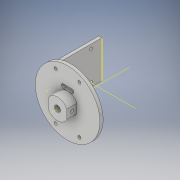
# Autodesk Inventor part: LidarLiteV3Mount
Saved by Autodesk Inventor 2019 (Build 230136000, 136)
## iProperties
Created: 2018-05-20
Part Number: LidarLiteV3Mount
Material: Generic
Document SubType Name: Modeling
Designer: samps
Density: 1 g/cm^3
Appearance: Default
Author: samps
Autodesk Inventor part; units mm, degrees
ref_plane "YZ Plane" through (0, 0, 0) normal (1, 0, 0) x (0, 1, 0)
ref_plane "XZ Plane" through (0, 0, 0) normal (0, 1, 0) x (-1, 0, 0)
ref_plane "XY Plane" through (0, 0, 0) normal (0, 0, 1) x (1, 0, 0)
sketch "Sketch1" plane through (0, 0, 0) normal (0, 0, 1) x (1, 0, 0)
  circle A0 centre (0, 0) radius 10
  dimension "d0" = 20
  constraints: 1 centre point, 1 coincident
  measures "d0" diameter of A0
extrude "Extrusion1" add sketch "Sketch1" along normal blind 10
sketch "Sketch2" plane through (0, 0, 10) normal (0, 0, 1) x (1, 0, 0)
  point P0 (0, 0)
  point P1 (0, 0)
  constraints: 1 coincident
hole "Hole1" at (0, 0, 10) direction (0, 0, -1) diameter 5 end through all
chamfer "Chamfer1" distance 0.5 angle 45 1 edges at (0, 2.5, 10)
sketch "Sketch3" plane through (0, 0, 10) normal (0, 0, 1) x (1, 0, 0)
  circle A0 centre (0, 0) radius 10 projected
  line L0 (-10, 0) -> (-9, 0)
  line L1 (-9, 0) -> (-9, 4.3589)
  line L2 (-9, 4.3589) -> (-10, 4.3589)
  line L3 (-10, 4.3589) -> (-10, 0)
  line L4 (-10, 0) -> (-9, 0)
  line L5 (-9, 0) -> (-9, -4.4002)
  line L6 (-9, -4.4002) -> (-10, -4.4002)
  line L7 (-10, -4.4002) -> (-10, 0)
  line L8 (10.026, 0) -> (9.026, 0)
  line L9 (9.026, 0) -> (9.026, 4.3589)
  line L10 (9.026, 4.3589) -> (10.026, 4.3589)
  line L11 (10.026, 4.3589) -> (10.026, 0)
  line L12 (10.026, 0) -> (9.026, 0)
  line L13 (9.026, 0) -> (9.026, -4.4002)
  line L14 (9.026, -4.4002) -> (10.026, -4.4002)
  line L15 (10.026, -4.4002) -> (10.026, 0)
  dimension "d13" = 1
  dimension "d14" = 1
  dimension "d15" = 1
  constraints: 32 end point, 8 parallel, 4 horizontal, 4 perpendicular, 4 point on line, 2 point on circle
  measures "d13" distance of L2.end L1.end
  measures "d14" distance of L5.end L6.end
  measures "d15" distance of L9.end L10.end
extrude "Extrusion2" cut sketch "Sketch3" against normal blind 10 contours L1 L0 A0 | L0 L5 A0 | A0 L5 L6 L7 | L9 L10 L11 L8 A0 | A0 L8 L9 | L8 L15 L14 L13 A0 | A0 L13 L8
sketch "Sketch4" plane through (9.026, -4.3048, 10) normal (1, 0, 0) x (0, 0, -1)
  line L0 (10, 4.3048) -> (5, 4.3048)
  line L1 (0.5, 1.8048) -> (0.5, 6.8048) projected
  dimension "d18" = 5
  constraints: 2 end point, 1 perpendicular
  measures "d18" distance of L0.start L0.end
hole "Hole2" at (9.026, 0, 5) direction (-1, 0, 0) diameter 3 end through all
sketch "Sketch5" plane through (9.026, -4.3048, 10) normal (1, 0, 0) x (0, 0, -1)
  circle A0 centre (5, 4.3048) radius 1.5 projected
  point P0 (10, 4.3048)
  constraints: 1 coincident
hole "Hole3" at (9.026, 0, 5) direction (-1, 0, 0) diameter 3.5 depth 3.5
sketch "Sketch6" plane through (-9, -4.3589, 10) normal (-1, 0, 0) x (0, 0, 1)
  circle A0 centre (-5, 4.3589) radius 1.5 projected
  point P0 (-10, 4.3589)
  constraints: 1 coincident
hole "Hole4" at (-9, 0, 5) direction (1, 0, 0) diameter 3.5 depth 3.5
sketch "Sketch7" plane through (0, 0, 0) normal (0, 0, -1) x (-1, 0, 0)
  line L0 (0, 0) -> (-9.026, 0)
  line L1 (-9.026, 0) -> (-9.026, 18)
  line L2 (-9.026, 18) -> (0, 18)
  line L3 (0, 18) -> (0, 0)
  line L4 (0, 0) -> (-9.026, 0)
  line L5 (-9.026, 0) -> (-9.026, -18)
  line L6 (-9.026, -18) -> (0, -18)
  line L7 (0, -18) -> (0, 0)
  line L8 (0, 18) -> (23, 18)
  line L9 (23, 18) -> (23, -18)
  line L10 (23, -18) -> (0, -18)
  line L11 (0, -18) -> (0, 18)
  dimension "d40" = 9.026
  dimension "d41" = 18
  dimension "d42" = 18
  dimension "d43" = 23
  constraints: 24 end point, 6 parallel, 3 horizontal, 3 perpendicular, 2 point on line
  measures "d40" distance of L1.end L2.end
  measures "d41" distance of L0.end L1.end
  measures "d42" distance of L5.end L4.end
  measures "d43" distance of L9.end L10.end
extrude "Extrusion3" add sketch "Sketch7" along normal blind 3
sketch "Sketch8" plane through (0, 0, -3) normal (0, 0, -1) x (-1, 0, 0)
  line L0 (23, 18) -> (-9.026, 18) projected
  line L1 (-9.026, -18) -> (23, -18) projected
  line L2 (23, 18) -> (20, 18)
  line L3 (20, 18) -> (20, -18)
  line L4 (20, -18) -> (23, -18)
  line L5 (23, -18) -> (23, 18)
  point P0 (0, 0)
  dimension "d46" = 3
  constraints: 8 end point, 2 parallel, 1 horizontal, 1 perpendicular, 1 point on line
  measures "d46" distance of L4.end L3.end
extrude "Extrusion4" add sketch "Sketch8" along normal blind 50
sketch "Sketch9" plane through (-20, -18, -3) normal (1, 0, 0) x (0, 0, -1)
  line L0 (0, 0) -> (0, 36) projected
  line L1 (0, 36) -> (25, 36)
  line L2 (-3, 36) -> (50, 36) projected
  line L3 (25, 36) -> (25, 18)
  line L4 (-3, 0) -> (50, 0) projected
  line L5 (25, 18) -> (39.5, 18)
  line L6 (39.5, 18) -> (39.5, 31.9)
  line L7 (39.5, 31.9) -> (25, 31.9)
  line L8 (25, 31.9) -> (25, 18)
  line L9 (25, 18) -> (39.5, 18)
  line L10 (39.5, 18) -> (39.5, 4.1)
  line L11 (39.5, 4.1) -> (25, 4.1)
  line L12 (25, 4.1) -> (25, 18)
  line L13 (25, 18) -> (10.5, 18)
  line L14 (10.5, 18) -> (10.5, 31.9)
  line L15 (10.5, 31.9) -> (25, 31.9)
  line L16 (25, 31.9) -> (25, 18)
  line L17 (25, 18) -> (10.5, 18)
  line L18 (10.5, 18) -> (10.5, 4.1)
  line L19 (10.5, 4.1) -> (25, 4.1)
  line L20 (25, 4.1) -> (25, 18)
  point P0 (-3, 18)
  dimension "d49" = 25
  dimension "d50" = 18
  dimension "d51" = 14.5
  dimension "d52" = 13.9
  dimension "d53" = 13.9
  dimension "d54" = 14.5
  constraints: 36 end point, 8 parallel, 5 perpendicular, 5 point on line, 4 horizontal
  measures "d49" distance of L0.end L1.end
  measures "d50" distance of L1.end L3.end
  measures "d51" distance of L7.end L6.end
  measures "d52" distance of L6.end L5.end
  measures "d53" distance of L9.end L10.end
  measures "d54" distance of L14.end L15.end
hole "Hole5" at (-20, 13.9, -13.5) at (-20, 13.9, -42.5) at (-20, -13.9, -42.5) at (-20, -13.9, -13.5) direction (-1, 0, 0) diameter 3 end through all
sketch "Sketch10" plane through (0, 0, -3) normal (0, 0, -1) x (-1, 0, 0)
  line L0 (-9.026, -18) -> (23, -18) projected
  circle A0 centre (0, 0) radius 29.2062
  circle A1 centre (0, 0) radius 2.5 projected
  circle A2 centre (0, 0) radius 31.206
  dimension "d62" = 62.412
  constraints: 2 coincident, 1 centre point, 3 other
  measures "d62" diameter of A2
extrude "Extrusion5" add sketch "Sketch10" against normal blind 3.175 contours A0 | A2
sketch "Sketch11" plane through (0, 0, -3) normal (0, 0, -1) x (-1, 0, 0)
  line L0 (23, -18) -> (23, 18) projected
  circle A0 centre (0, 0) radius 29.2062
  line L1 (23, 18) -> (-23, 18)
  line L2 (-23, 18) -> (-23, -18)
  line L3 (-23, -18) -> (23, -18)
  line L4 (23, -18) -> (23, 18)
  circle A1 centre (0, 0) radius 2.5 projected
  line L5 (0, 0) -> (0, 23)
  line L6 (0, 23) -> (11.5, 23)
  line L7 (11.5, 23) -> (-11.5, 23)
  line L8 (-11.5, 23) -> (-11.5, -23)
  line L9 (-11.5, -23) -> (11.5, -23)
  line L10 (11.5, -23) -> (11.5, 23)
  dimension "d65" = 23
  dimension "d66" = 11.5
  dimension "d67" = 23
  dimension "d68" = 46
  constraints: 20 end point, 4 parallel, 4 perpendicular, 2 horizontal, 2 point on circle, 1 centre point, 1 coincident
  measures "d65" distance of L5.start L5.end
  measures "d66" distance of L5.end L6.end
  measures "d67" distance of L9.end L8.end
  measures "d68" distance of L8.end L7.end
hole "Hole6" at (11.5, 23, -3) at (-11.5, 23, -3) at (11.5, -23, -3) at (-11.5, -23, -3) direction (0, 0, 1) diameter 3 depth 3.5
sketch "Sketch12" plane through (-20, -18, -3) normal (1, 0, 0) x (0, 0, -1)
  line L0 (0, 0) -> (0, 36) projected
  line L1 (50, 0) -> (50, 36) projected
  point P0 (-3, 18)
  point P1 (25, 18)
sketch "Sketch13" plane through (0, 0, 0.175) normal (0, 0, 1) x (1, 0, 0)
  arc A0 (9.026, 4.3048) -> (-9, 4.3589) centre (0, 0) ccw projected
  line L0 (0, 10) -> (6, 10)
  line L1 (6, 10) -> (6, 14)
  line L2 (6, 14) -> (0, 14)
  line L3 (0, 14) -> (0, 10)
  line L4 (6, 14) -> (-6, 14)
  line L5 (-6, 14) -> (-6, 10)
  line L6 (-6, 10) -> (6, 10)
  line L7 (6, 10) -> (6, 14)
  dimension "d76" = 6
  dimension "d77" = 4
  dimension "d78" = 12
  constraints: 16 end point, 4 parallel, 2 horizontal, 2 perpendicular, 1 point on circle, 1 point on line
  measures "d76" distance of L2.end L1.end
  measures "d77" distance of L1.end L0.end
  measures "d78" distance of L6.end L5.end
extrude "Extrusion6" cut sketch "Sketch13" against normal blind 3.175
fillet "Fillet1" radius 2 4 edges at (-6, 14, -1.4125) (6, 14, -1.4125) (6, 10, -1.4125) (-6, 10, -1.4125)
sketch "Sketch14" plane through (-23, -18, -3) normal (-1, 0, 0) x (0, 0, 1)
  circle A0 centre (-39.5, 31.9) radius 1.5 projected
  circle A1 centre (-10.5, 4.1) radius 1.5 projected
  line L0 (-39.5, 31.9) -> (-10.5, 4.1)
  circle A2 centre (-39.5, 4.1) radius 1.5 projected
  line L1 (-10.5, 4.1) -> (-39.5, 4.1)
  circle A3 centre (-10.5, 31.9) radius 1.5 projected
  line L2 (-39.5, 4.1) -> (-10.5, 31.9)
  point P0 (3, 18)
  point P1 (-25, 18)
  constraints: 6 end point, 1 horizontal, 1 midpoint
hole "Hole7" at (-23, 0, -28) direction (1, 0, 0) diameter 5 end through all
body "Solid1"
